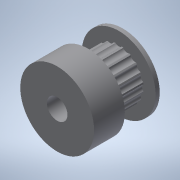
# Autodesk Inventor part: GT2 20T Drive Pulley
Saved by Autodesk Inventor 2022 (Build 260153000, 153)
## iProperties
Created: 2015-06-17
Part Number: GT2 20T Drive Pulley
Material: Generic
Document SubType Name: Modeling
Designer: Andrew
Density: 1 g/cm^3
Appearance: Default
Author: Andrew
Autodesk Inventor part; units mm, degrees
ref_plane "YZ Plane" through (0, 0, 0) normal (1, 0, 0) x (0, 1, 0)
ref_plane "XZ Plane" through (0, 0, 0) normal (0, 1, 0) x (-1, 0, 0)
ref_plane "XY Plane" through (0, 0, 0) normal (0, 0, 1) x (1, 0, 0)
sketch "Sketch1" plane through (0, 0, 0) normal (0, 0, 1) x (1, 0, 0)
  line L0 (0, 0) -> (0, 16) construction
  line L1 (0, 16) -> (2.5, 16) construction
  line L2 (2.5, 16) -> (9, 16)
  line L3 (9, 16) -> (9, 15)
  line L4 (9, 15) -> (6.1, 15)
  line L5 (6.1, 15) -> (6.1, 7.5)
  line L6 (6.1, 7.5) -> (9, 7.5)
  line L7 (9, 7.5) -> (9, 0)
  line L8 (9, 0) -> (2.5, 0)
  line L9 (2.5, 0) -> (2.5, 16)
  dimension "d0" = 2.5
  dimension "d1" = 7.5
  dimension "d2" = 7.5
  dimension "d3" = 9
  dimension "d4" = 1
  dimension "d6" = 6.1
  constraints: 20 end point, 5 perpendicular, 4 point on line, 1 horizontal, 1 parallel, 1 vertical
  measures "d0" distance between parallel lines of L0 L9
  measures "d1" distance of L4.end L5.end
  measures "d2" distance of L6.end L7.end
  measures "d3" distance between parallel lines of L0 L7
  measures "d4" distance between parallel lines of L2 L4
  measures "d6" distance between parallel lines of L0 L5
revolve "Revolution1" add sketch "Sketch1" angle 360 about axis through (0, 0, 0) along (0, 1, 0)
sketch "Sketch2" plane through (0, 7.5, 0) normal (0, 1, 0) x (1, 0, 0)
  line L0 (0, 0) -> (0, -6.7)
  circle A0 centre (0, -6.7) radius 1
  dimension "d8" = 2
  dimension "d9" = 6.7
  constraints: 2 end point, 1 centre point, 1 coincident, 1 vertical
  measures "d8" diameter of A0
  measures "d9" distance of L0.start L0.end
extrude "Extrusion1" cut sketch "Sketch2" along normal up to surface (7.5 mm away)
pattern_circular "Circular Pattern1" count 20 over 360 about axis through (0, 11.25, 0) along (0, -1, 0) of "Extrusion1"
body "Solid1"
